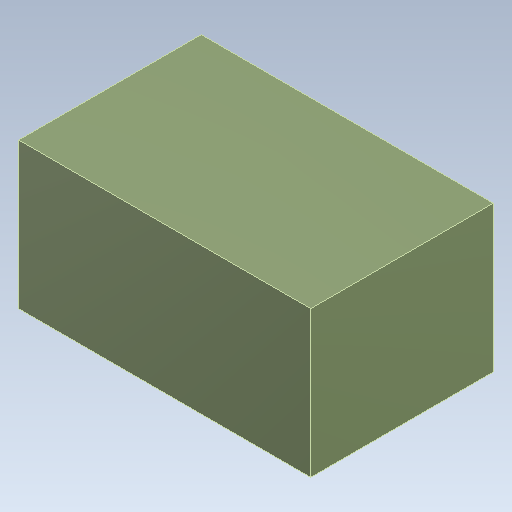
# Autodesk Inventor part: 1UF
Saved by Autodesk Inventor 2021 (Build 250183000, 183)
## iProperties
Created: 2020-11-03
Part Number: 1UF
Material: Generic
Document SubType Name: Modeling
Designer: faiya
Density: 1 g/cm^3
Appearance: C0603K, 1UF
Author: faiya
Autodesk Inventor part; units mm, degrees
ref_plane "YZ Plane" through (0, 0, 0) normal (1, 0, 0) x (0, 1, 0)
ref_plane "XZ Plane" through (0, 0, 0) normal (0, 1, 0) x (-1, 0, 0)
ref_plane "XY Plane" through (0, 0, 0) normal (0, 0, 1) x (1, 0, 0)
sketch "C0603K, 1UF_13" plane through (0, 0, 0) normal (0, 0, 1) x (1, 0, 0)
  line L0 (-0.8, 0.4008) -> (0.8, 0.4008)
  line L1 (0.8, 0.4008) -> (0.8, -0.4)
  line L2 (0.8, -0.4) -> (-0.8, -0.4)
  line L3 (-0.8, -0.4) -> (-0.8, 0.4008)
  constraints: 8 end point
extrude "Extrusion1" add sketch "C0603K, 1UF_13" along normal blind 1
body "Solid1"
